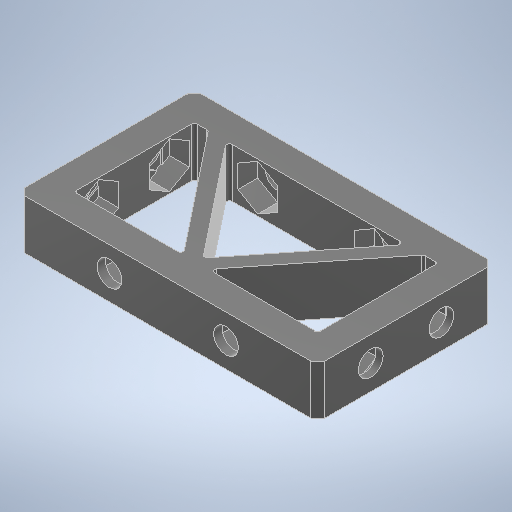
# Autodesk Inventor part: 3D_club-fix
Saved by Autodesk Inventor 2025 (Build 290162000, 162)
## iProperties
Created: 2024-07-27
Part Number: 3D_club-fix
Material: 一般
Document SubType Name: Modeling
Designer: 8326d
Density: 1 g/cm^3
Appearance: 滑らか - 黒
Author: 8326d
## iProperties of the stored document 3D_club-fix_3D プリント.ipt
Created: 2024-08-04
Part Number: 3D_club-fix_3D プリント
Material: 一般
Document SubType Name: Modeling
Designer: 8326d
Density: 1 g/cm^3
Appearance: 既定
Author: 8326d
Autodesk Inventor part; units mm, degrees
ref_plane "YZ Plane" through (0, 0, 0) normal (1, 0, 0) x (0, 1, 0)
ref_plane "XZ Plane" through (0, 0, 0) normal (0, 1, 0) x (-1, 0, 0)
ref_plane "XY Plane" through (0, 0, 0) normal (0, 0, 1) x (1, 0, 0)
sketch "スケッチ1" plane through (0, 0, 0) normal (0, 0, 1) x (1, 0, 0)
  line L0 (-21.25, -3.5) -> (21.25, -3.5)
  line L1 (21.25, -3.5) -> (21.25, 3.5)
  line L2 (21.25, 3.5) -> (-21.25, 3.5)
  line L3 (-21.25, 3.5) -> (-21.25, -3.5)
  line L4 (-21.25, -3.5) -> (21.25, 3.5) construction
  line L5 (21.25, -3.5) -> (-21.25, 3.5) construction
  point P0 (0, 0)
  dimension "d0" = 42.5
  dimension "d1" = 7
  constraints: 12 end point, 2 midpoint, 2 parallel, 1 horizontal, 1 perpendicular
  measures "d0" distance of L2.end L1.end
  measures "d1" distance of L1.end L0.end
extrude "押し出し1" add sketch "スケッチ1" along normal mid plane 25
sketch "スケッチ2" plane through (0, 0, 12.5) normal (0, 0, 1) x (1, 0, 0)
  line L0 (-21.25, 3.5) -> (-21.25, -3.5) projected
  line L1 (21.25, -3.5) -> (21.25, 3.5) projected
  line L2 (-21.25, 0) -> (21.25, 0) construction
  point P0 (0, 0)
  point P1 (-8.25, 0)
  point P2 (8.25, 0)
  point P3 (0, 0)
  dimension "d4" = 16.5
  dimension "d5" = 8.25
  constraints: 3 midpoint, 2 end point, 2 point on line
  measures "d4" distance of point (8.25, 0) point (-8.25, 0)
  measures "d5" distance of point (-8.25, 0) point (0, 0)
hole "穴1" at (-8.25, 0, 12.5) at (8.25, 0, 12.5) direction (0, 0, -1) diameter 3.5 end through all
sketch "スケッチ3" plane through (-21.25, 3.5, 12.5) normal (0, 1, 0) x (1, 0, 0)
  line L0 (0, 25) -> (0, 0) projected
  line L1 (42.5, 25) -> (42.5, 0) projected
  line L2 (0, 12.5) -> (42.5, 12.5) construction
  line L3 (38.5, 4) -> (4, 4)
  line L4 (4, 4) -> (4, 21)
  line L5 (4, 21) -> (38.5, 21)
  line L6 (38.5, 21) -> (38.5, 4)
  line L7 (38.5, 4) -> (4, 21) construction
  line L8 (4, 4) -> (38.5, 21) construction
  line L9 (42.5, 0) -> (0, 0) projected
  point P0 (21.25, 12.5)
  dimension "d13" = 4
  dimension "d14" = 4
  constraints: 14 end point, 4 midpoint, 2 parallel, 1 horizontal, 1 perpendicular
  measures "d13" distance between parallel lines of L9 L3
  measures "d14" distance between parallel lines of L0 L4
extrude "押し出し2" cut sketch "スケッチ3" against normal through all
sketch "スケッチ4" plane through (17.25, 3.5, 8.5) normal (0, 0, -1) x (-1, 0, 0)
  circle A0 centre (25.5, -3.5) radius 1.75 projected
  circle A1 centre (9, -3.5) radius 1.75 projected
  line L0 (25.5, -0.2668) -> (28.3, -1.8834)
  line L1 (28.3, -1.8834) -> (28.3, -5.1166)
  line L2 (28.3, -5.1166) -> (25.5, -6.7332)
  line L3 (25.5, -6.7332) -> (22.7, -5.1166)
  line L4 (22.7, -5.1166) -> (22.7, -1.8834)
  line L5 (22.7, -1.8834) -> (25.5, -0.2668)
  circle A2 centre (9, -3.5) radius 1.75 projected
  line L6 (9, -0.2668) -> (11.8, -1.8834)
  line L7 (11.8, -1.8834) -> (11.8, -5.1166)
  line L8 (11.8, -5.1166) -> (9, -6.7332)
  line L9 (9, -6.7332) -> (6.2, -5.1166)
  line L10 (6.2, -5.1166) -> (6.2, -1.8834)
  line L11 (6.2, -1.8834) -> (9, -0.2668)
  point P0 (17.25, -3.5)
  point P1 (22.7, -3.5)
  dimension "d17" = 5.6
  dimension "d18" = 5.6
  constraints: 24 end point, 2 coincident, 2 vertical alignment, 1 midpoint, 26 other
  measures "d17" distance from line of point (22.7, -3.5) L1
  measures "d18" distance between parallel lines of L10 L7
extrude "押し出し3" cut sketch "スケッチ4" against normal blind 2.8
sketch "スケッチ5" plane through (-21.25, -3.5, 12.5) normal (-1, 0, 0) x (0, 0, 1)
  line L0 (0, 7) -> (0, 0) projected
  line L1 (-25, 0) -> (-25, 7) projected
  line L2 (0, 3.5) -> (-25, 3.5) construction
  point P0 (-12.5, 3.5)
  point P1 (-7.5, 3.5)
  point P2 (-17.5, 3.5)
  point P3 (-12.5, 3.5)
  dimension "d21" = 5
  dimension "d22" = 5
  constraints: 3 midpoint, 2 end point, 2 point on line
  measures "d21" distance of point (-12.5, 3.5) point (-7.5, 3.5)
  measures "d22" distance of point (-12.5, 3.5) point (-17.5, 3.5)
hole "穴2" at (-21.25, 0, 5) at (-21.25, 0, -5) direction (1, 0, 0) diameter 3.5 end through all
sketch "スケッチ6" plane through (17.25, 3.5, -8.5) normal (-1, 0, 0) x (0, 0, 1)
  circle A0 centre (13.5, -3.5) radius 1.75 projected
  circle A1 centre (3.5, -3.5) radius 1.75 projected
  circle A2 centre (13.5, -3.5) radius 1.75 projected
  line L0 (13.5, -6.7332) -> (10.7, -5.1166)
  line L1 (10.7, -5.1166) -> (10.7, -1.8834)
  line L2 (10.7, -1.8834) -> (13.5, -0.2668)
  line L3 (13.5, -0.2668) -> (16.3, -1.8834)
  line L4 (16.3, -1.8834) -> (16.3, -5.1166)
  line L5 (16.3, -5.1166) -> (13.5, -6.7332)
  line L6 (3.5, -6.7332) -> (0.7, -5.1166)
  line L7 (0.7, -5.1166) -> (0.7, -1.8834)
  line L8 (0.7, -1.8834) -> (3.5, -0.2668)
  line L9 (3.5, -0.2668) -> (6.3, -1.8834)
  line L10 (6.3, -1.8834) -> (6.3, -5.1166)
  line L11 (6.3, -5.1166) -> (3.5, -6.7332)
  point P0 (8.5, -3.5)
  dimension "d30" = 5.6
  dimension "d31" = 5.6
  constraints: 24 end point, 2 coincident, 2 vertical alignment, 26 other
  measures "d30" distance between parallel lines of L1 L4
  measures "d31" distance between parallel lines of L7 L10
extrude "押し出し4" cut sketch "スケッチ6" against normal blind 3
sketch "スケッチ7" plane through (20.25, 3.5, -8.5) normal (-1, 0, 0) x (0, 0, 1)
  line L0 (16.3, -1.8834) -> (16.3, -5.1166) projected
  line L1 (13.5, -0.2668) -> (16.3, -1.8834) projected
  line L2 (10.7, -1.8834) -> (13.5, -0.2668) projected
  line L3 (10.7, -5.1166) -> (10.7, -1.8834) projected
  line L4 (13.5, -6.7332) -> (10.7, -5.1166) projected
  line L5 (16.3, -5.1166) -> (13.5, -6.7332) projected
  circle A0 centre (13.5, -3.5) radius 1.75 projected
  line L6 (6.3, -1.8834) -> (6.3, -5.1166) projected
  line L7 (3.5, -0.2668) -> (6.3, -1.8834) projected
  line L8 (0.7, -1.8834) -> (3.5, -0.2668) projected
  line L9 (0.7, -5.1166) -> (0.7, -1.8834) projected
  line L10 (3.5, -6.7332) -> (0.7, -5.1166) projected
  line L11 (6.3, -5.1166) -> (3.5, -6.7332) projected
  circle A1 centre (3.5, -3.5) radius 1.75 projected
  line L12 (15.25, -5.7228) -> (15.25, -1.2772)
  line L13 (14.55, -6.1269) -> (10.7, -3.9041)
  line L14 (10.7, -3.0959) -> (14.55, -0.8731)
  line L15 (13.5, -0.2668) -> (16.3, -1.8834) projected
  line L16 (10.7, -5.1166) -> (10.7, -1.8834) projected
  circle A2 centre (13.5, -3.5) radius 1.75 projected
  point P0 (8.5, -3.5)
  constraints: 6 end point, 6 point on line, 3 parallel, 3 tangent
extrude "押し出し5" add sketch "スケッチ7" along normal blind 0.2 contours L0 L5 L12 L1 | L14 L3 L2 L1 | L5 L4 L3 L13
mirror "ミラー1" about plane through (0, 0, 0) normal (0, 0, 1) of "押し出し3", "押し出し5"
mirror "ミラー2" about plane through (0, 0, 0) normal (1, 0, 0) of "押し出し4", "押し出し3", "押し出し5", "ミラー1"
chamfer "面取り1" distance 1 angle 45 4 edges at (-21.25, 0, 12.5) (21.25, 0, 12.5) (21.25, 0, -12.5) (-21.25, 0, -12.5)
sketch "スケッチ8" plane through (-20.25, 3.5, 12.5) normal (0, 1, 0) x (1, 0, 0)
  line L0 (3, 21) -> (37.5, 21) projected
  line L1 (37.5, 4) -> (3, 4) projected
  line L2 (3, 4) -> (3, 21) projected
  line L3 (5, 21) -> (19.4665, 2.7573)
  line L4 (19.4665, 2.7573) -> (21.0335, 4)
  line L5 (21.0335, 4) -> (6.5671, 22.2427)
  line L6 (6.5671, 22.2427) -> (5, 21)
  point P0 (20.25, 12.5)
  point P1 (20.25, 3.3787)
  point P2 (20.25, 4)
  point P3 (7.5525, 21)
  point P4 (18.481, 4)
  dimension "d40" = 2
  dimension "d47" = 2
  constraints: 8 end point, 2 midpoint, 2 parallel, 2 point on line, 1 perpendicular, 1 vertical alignment
  measures "d40" distance between parallel lines of L5 L3
  measures "d47" distance from line of L2 L3.start
extrude "押し出し6" add sketch "スケッチ8" against normal up to surface (7 mm away) contours L6 L5 L0 | L0 L5 L1 L3 | L1 L4 L3
mirror "ミラー3" about plane through (0, 0, 0) normal (1, 0, 0) of "押し出し6"
fillet "フィレット2" radius 0.4 11 edges at (-1.769, 0, 8.5) (0, 0, 7.5119) (1.769, 0, 8.5) (-17.25, 0, 8.5) (-12.6975, 0, -8.5) (12.6975, 0, -8.5) (17.25, 0, 8.5) (-17.25, 0, -8.5) (17.25, 0, -8.5) (-15.25, 0, -8.5) (15.25, 0, -8.5)
equation "\"d5\" = 0.5 * d4"
equation "\"d18\" = d17"
equation "\"d22\" = d21"
equation "\"d31\" = d30"
